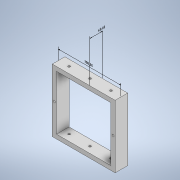
# Autodesk Inventor part: IdeaBase
Saved by Autodesk Inventor 2021 (Build 250183000, 183)
## iProperties
Created: 2022-05-21
Part Number: IdeaBase
Material: Genérico
Document SubType Name: Modeling
Designer: 79449
Density: 1 g/cm^3
Appearance: Valor por defecto
Author: 79449
Autodesk Inventor part; units mm, degrees
ref_plane "YZ Plane" through (0, 0, 0) normal (1, 0, 0) x (0, 1, 0)
ref_plane "XZ Plane" through (0, 0, 0) normal (0, 1, 0) x (-1, 0, 0)
ref_plane "XY Plane" through (0, 0, 0) normal (0, 0, 1) x (1, 0, 0)
sketch "Boceto1" plane through (0, 0, 0) normal (0, 0, 1) x (1, 0, 0)
  line L0 (-150, 150) -> (150, 150)
  line L1 (150, 150) -> (150, -150)
  line L2 (150, -150) -> (-150, -150)
  line L3 (-150, -150) -> (-150, 150)
  line L4 (-150, 150) -> (150, -150) construction
  line L5 (150, 150) -> (-150, -150) construction
  line L6 (130, -130) -> (-130, -130)
  line L7 (-130, -130) -> (-130, 130)
  line L8 (-130, 130) -> (130, 130)
  line L9 (130, 130) -> (130, -130)
  line L10 (130, -130) -> (-130, 130) construction
  line L11 (-130, -130) -> (130, 130) construction
  point P0 (0, 0)
  dimension "d2" = 300
  dimension "d3" = 300
  dimension "d20" = 20
  constraints: 24 end point, 4 midpoint, 4 parallel, 2 horizontal, 2 perpendicular, 1 point on line
  measures "d2" distance of L1.end L2.end
  measures "d3" distance of L0.end L1.end
  measures "d20" distance between parallel lines of L9 L1
extrude "Extrusión1" add sketch "Boceto1" along normal blind 60
sketch "Boceto3" plane through (-150, -150, 0) normal (0, -1, 0) x (1, 0, 0)
  circle A0 centre (150, 30) radius 5
  line L0 (0, 60) -> (300, 60) projected
  line L1 (0, 0) -> (0, 60) projected
  line L2 (20, 60) -> (280, 60) projected
  line L3 (150, 60) -> (150, 0) construction
  circle A1 centre (250, 30) radius 5
  circle A2 centre (50, 30) radius 5
  dimension "d21" = 10
  dimension "d24" = 30
  dimension "d25" = 150
  dimension "d26" = 10
  dimension "d27" = 30
  dimension "d28" = 100
  dimension "d29" = 10
  dimension "d30" = 100
  dimension "d31" = 30
  constraints: 3 centre point, 2 end point, 1 midpoint, 1 perpendicular
  measures "d21" diameter of A0
  measures "d24" distance from line of A0.centre L0
  measures "d25" distance from line of L1 A0.centre
  measures "d26" diameter of A1
  measures "d27" distance from line of L0 A1.centre
  measures "d28" distance of A0.centre A1.centre
  measures "d29" diameter of A2
  measures "d30" distance of A0.centre A2.centre
  measures "d31" distance from line of L0 A2.centre
extrude "Extrusión3" cut sketch "Boceto3" against normal up to surface (300 mm away)
sketch "Boceto4" plane through (0, 0, 60) normal (0, 0, 1) x (1, 0, 0)
  circle A0 centre (-140, 0) radius 5
  line L0 (-130, -130) -> (-130, 130) projected
  line L1 (-150, -150) -> (150, -150) projected
  circle A1 centre (140, 0) radius 5
  line L2 (130, 130) -> (130, -130) projected
  point P0 (0, 0)
  dimension "d32" = 10
  dimension "d33" = 10
  dimension "d34" = 150
  dimension "d35" = 10
  dimension "d36" = 150
  dimension "d37" = 10
  constraints: 2 centre point
  measures "d32" diameter of A0
  measures "d33" distance from line of L0 A0.centre
  measures "d34" distance from line of L1 A0.centre
  measures "d35" distance from line of L2 A1.centre
  measures "d36" distance from line of L1 A1.centre
  measures "d37" diameter of A1
extrude "Extrusión4" cut sketch "Boceto4" against normal through all
